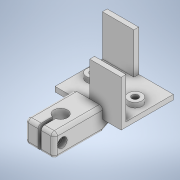
# Autodesk Inventor part: linearGuideMount
Saved by Autodesk Inventor 2020 (Build 240168000, 168)
## iProperties
Created: 2020-01-08
Part Number: linearGuideMount
Material: Generic
Document SubType Name: Modeling
Designer: PAB
Density: 1 g/cm^3
Appearance: Default
Author: PAB
Autodesk Inventor part; units mm, degrees
ref_plane "YZ Plane" through (0, 0, 0) normal (1, 0, 0) x (0, 1, 0)
ref_plane "XZ Plane" through (0, 0, 0) normal (0, 1, 0) x (-1, 0, 0)
ref_plane "XY Plane" through (0, 0, 0) normal (0, 0, 1) x (1, 0, 0)
sketch "Sketch1" plane through (0, 0, 0) normal (0, 1, 0) x (-1, 0, 0)
  line L0 (20.5, 16.2) -> (-20.5, 16.2)
  line L1 (-20.5, 16.2) -> (-20.5, -16.2)
  line L2 (-20.5, -16.2) -> (20.5, -16.2)
  line L3 (20.5, -16.2) -> (20.5, 16.2)
  point P0 (0, 0)
  dimension "d0" = 41
  dimension "d1" = 32.4
  constraints: 8 end point, 2 parallel, 1 horizontal, 1 perpendicular
  measures "d0" distance of L2.end L1.end
  measures "d1" distance of L1.end L0.end
extrude "Extrusion1" add sketch "Sketch1" along normal blind 3
sketch "Sketch3" plane through (0, 3, 0) normal (0, 1, 0) x (1, 0, 0)
  line L0 (-20.5, -16.2) -> (20.5, -16.2) projected
  line L1 (-20.5, 16.2) -> (-20.5, -16.2) projected
  line L2 (20.5, -16.2) -> (-20.5, -16.2)
  line L3 (-20.5, -16.2) -> (-20.5, -13.2)
  line L4 (-20.5, -13.2) -> (20.5, -13.2)
  line L5 (20.5, -13.2) -> (20.5, -16.2)
  line L6 (20.5, 16.2) -> (-20.5, 16.2) projected
  line L7 (20.5, 16.2) -> (-20.5, 16.2)
  line L8 (-20.5, 16.2) -> (-20.5, 13.2)
  line L9 (-20.5, 13.2) -> (20.5, 13.2)
  line L10 (20.5, 13.2) -> (20.5, 16.2)
  point P0 (0, 0)
  dimension "d8" = 3
  dimension "d9" = 3
  constraints: 16 end point, 4 parallel, 2 horizontal, 2 perpendicular, 2 point on line
  measures "d8" distance of L2.end L3.end
  measures "d9" distance of L8.end L7.end
extrude "Extrusion3" add sketch "Sketch3" along normal blind 25.4
sketch "Sketch4" plane through (20.5, 0, -16.2) normal (0, 0, -1) x (-1, 0, 0)
  line L0 (41, 3) -> (0, 3) projected
  line L1 (0, 28.4) -> (41, 28.4) projected
  line L2 (0, 3) -> (21.5, 3)
  line L3 (21.5, 3) -> (21.5, 28.4)
  line L4 (21.5, 28.4) -> (0, 28.4)
  line L5 (0, 28.4) -> (0, 3)
  point P0 (20.5, 0)
  dimension "d12" = 21.5
  constraints: 8 end point, 2 parallel, 1 horizontal, 1 perpendicular, 1 point on line
  measures "d12" distance of L4.end L3.end
extrude "Extrusion4" cut sketch "Sketch4" against normal blind 3
sketch "Sketch5" plane through (-20.5, 0, 16.2) normal (0, 0, 1) x (1, 0, 0)
  line L0 (41, 28.4) -> (0, 28.4) projected
  line L1 (19.5, 3) -> (41, 3) projected
  line L2 (0, 28.4) -> (21.5, 28.4)
  line L3 (21.5, 28.4) -> (21.5, 3)
  line L4 (21.5, 3) -> (0, 3)
  line L5 (0, 3) -> (0, 28.4)
  point P0 (20.5, 0)
  dimension "d15" = 21.5
  constraints: 8 end point, 2 parallel, 1 horizontal, 1 perpendicular, 1 point on line
  measures "d15" distance of L3.end L4.end
extrude "Extrusion5" cut sketch "Sketch5" against normal blind 3
sketch "Sketch6" plane through (0, 3, 0) normal (0, 1, 0) x (1, 0, 0)
  circle A0 centre (13, 0) radius 4.25
  circle A1 centre (-13, 0) radius 4.25
  point P0 (0, 0)
  dimension "d20" = 8.5
  dimension "d21" = 8.5
  constraints: 2 centre point
  measures "d20" diameter of A0
  measures "d21" diameter of A1
extrude "Extrusion6" add sketch "Sketch6" along normal blind 3
sketch "Sketch7" plane through (0, 0, 0) normal (0, -1, 0) x (1, 0, 0)
  circle A0 centre (-13, 0) radius 4.25 projected
  circle A1 centre (-13, 0) radius 2
  circle A2 centre (13, 0) radius 4.25 projected
  circle A3 centre (13, 0) radius 2
  point P0 (0, 0)
  dimension "d24" = 4
  dimension "d25" = 4
  constraints: 2 centre point, 2 coincident
  measures "d24" diameter of A1
  measures "d25" diameter of A3
extrude "Extrusion7" cut sketch "Sketch7" against normal blind 6 contours A1 | A3
sketch "Sketch8" plane through (0, 0, 0) normal (0, -1, 0) x (1, 0, 0)
  circle A0 centre (-13, 0) radius 2 projected
  circle A1 centre (-13, 0) radius 3
  circle A2 centre (13, 0) radius 2 projected
  circle A3 centre (13, 0) radius 3
  point P0 (0, 0)
  dimension "d28" = 6
  dimension "d29" = 6
  constraints: 2 centre point, 2 coincident
  measures "d28" diameter of A1
  measures "d29" diameter of A3
extrude "Extrusion8" cut sketch "Sketch8" against normal blind 3 contours A0 | A1 | A2 | A3
sketch "Sketch9" plane through (-20.5, 0, 16.2) normal (0, 0, 1) x (1, 0, 0)
  line L0 (11.5, 7) -> (29.5, 7)
  line L1 (29.5, 7) -> (29.5, -7)
  line L2 (29.5, -7) -> (11.5, -7)
  line L3 (11.5, -7) -> (11.5, 7)
  point P0 (20.5, 0)
  dimension "d32" = 18
  dimension "d33" = 14
  constraints: 8 end point, 2 parallel, 1 horizontal, 1 perpendicular
  measures "d32" distance of L1.end L2.end
  measures "d33" distance of L0.end L1.end
extrude "Extrusion9" add sketch "Sketch9" along normal blind 30
sketch "Sketch10" plane through (0, 0, 0) normal (0, -1, 0) x (1, 0, 0)
  line L0 (9, 16.2) -> (20.5, 16.2) projected
  line L1 (9, 16.2) -> (6, 16.2)
  line L2 (6, 16.2) -> (6, 3)
  line L3 (6, 3) -> (9, 3)
  line L4 (9, 3) -> (9, 16.2)
  line L5 (1, 16.2) -> (-9, 16.2) projected
  line L6 (-9, 16.2) -> (-6, 16.2)
  line L7 (-6, 16.2) -> (-6, 3)
  line L8 (-6, 3) -> (-9, 3)
  line L9 (-9, 3) -> (-9, 16.2)
  point P0 (0, 0)
  dimension "d36" = 3
  dimension "d37" = 3
  constraints: 16 end point, 4 parallel, 2 horizontal, 2 perpendicular
  measures "d36" distance of L3.end L2.end
  measures "d37" distance of L7.end L8.end
extrude "Extrusion10" add sketch "Sketch10" along normal blind 7
sketch "Sketch11" plane through (-9, 3, 16.2) normal (-1, 0, 0) x (0, 0, 1)
  line L0 (0, -3) -> (-13.2, -3) projected
  line L1 (-13.2, -3) -> (0, -10)
  line L2 (-13.2, -10) -> (30, -10) projected
  line L3 (-13.2, -3) -> (-13.2, -10) projected
  line L4 (-13.2, -10) -> (-13.2, -3)
  point P0 (-16.2, -3)
  constraints: 4 end point, 1 collinear, 1 point on line
extrude "Extrusion11" cut sketch "Sketch11" against normal blind 18
sketch "Sketch12" plane through (-9, 7, 16.2) normal (0, 1, 0) x (1, 0, 0)
  circle A0 centre (9, -17) radius 4.25
  line L0 (18, -30) -> (0, -30) projected
  line L1 (8, -30) -> (10, -30)
  line L2 (10, -30) -> (10, -20.6375)
  line L3 (10, -20.6375) -> (8, -20.6375)
  line L4 (8, -20.6375) -> (8, -30)
  point P0 (9, 16.2)
  point P1 (10, -21.1307)
  point P2 (8, -21.1307)
  dimension "d42" = 8.5
  dimension "d43" = 2
  constraints: 8 end point, 2 parallel, 1 centre point, 1 horizontal, 1 perpendicular, 1 point on line
  measures "d42" diameter of A0
  measures "d43" distance of L3.end L2.end
extrude "Extrusion12" cut sketch "Sketch12" against normal blind 30
sketch "Sketch13" plane through (9, 0, 16.2) normal (1, 0, 0) x (0, 0, -1)
  circle A0 centre (-25, 0) radius 3
  point P0 (16.2, 0)
  dimension "d46" = 6
  constraints: 1 centre point
  measures "d46" diameter of A0
extrude "Extrusion13" cut sketch "Sketch13" against normal blind 3
mirror "Mirror1" about plane through (0, 0, 0) normal (1, 0, 0) of "Extrusion13"
sketch "Sketch14" plane through (9, 0, 16.2) normal (1, 0, 0) x (0, 0, -1)
  circle A0 centre (-25, 0) radius 3 projected
  circle A1 centre (-25, 0) radius 2
  point P0 (16.2, 0)
  dimension "d49" = 4
  constraints: 1 centre point, 1 coincident
  measures "d49" diameter of A1
extrude "Extrusion14" cut sketch "Sketch14" against normal blind 20 contours A1
fillet "Fillet1" radius 2 14 edges at (9, 0, 46.2) (9, 7, 31.2) (-9, 7, 31.2) (-5, 7, 46.2) (5, 7, 46.2) (5, -7, 46.2) (-5, -7, 46.2) (-9, 0, 46.2) (9, -7, 31.2) (-9, -7, 31.2) (9, -3.5, 9.6) (6, -3.5, 9.6) (-6, -3.5, 9.6) (-9, -3.5, 9.6)
fillet "Fillet2" radius 2 1 edges at (0, -7, 16.2)
body "Solid1"
